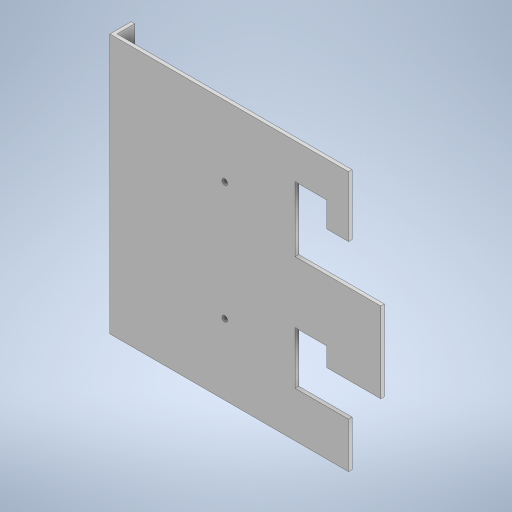
# Autodesk Inventor part: Coffee_Machine_Base
Saved by Autodesk Inventor 2023.5 (Build 275446020, 446B)
## iProperties
Created: 2025-04-17
Part Number: Coffee_Machine_Base
Material: Generic
Document SubType Name: Modeling
Designer: Lucky Sah
Density: 1 g/cm^3
Appearance: Default
Author: Lucky Sah
Autodesk Inventor part; units mm, degrees
ref_plane "YZ Plane" through (0, 0, 0) normal (1, 0, 0) x (0, 1, 0)
ref_plane "XZ Plane" through (0, 0, 0) normal (0, 1, 0) x (-1, 0, 0)
ref_plane "XY Plane" through (0, 0, 0) normal (0, 0, 1) x (1, 0, 0)
sketch "Sketch1" plane through (0, 0, 0) normal (0, 0, 1) x (1, 0, 0)
  line L0 (0, 0) -> (260, 0)
  line L1 (260, 0) -> (260, 125)
  line L2 (220, 147) -> (0, 147)
  line L3 (0, 147) -> (0, 0)
  circle A0 centre (240, 135) radius 8
  circle A1 centre (240, 135) radius 10
  line L4 (250, 135) -> (250.202, 135)
  line L5 (230, 135) -> (230, 137)
  arc A2 (230, 137) -> (220, 147) centre (220, 137) ccw
  line L6 (260, 147) -> (260, 147)
  line L7 (250, 135) -> (250, 137)
  line L8 (240, 125) -> (260, 125)
  line L9 (0, 73.5) -> (260, 73.5)
  line L10 (130, 112.7628) -> (117.7684, 112.7628)
  line L11 (99.8322, 119.3312) -> (99.8322, 90.3139)
  line L12 (99.8322, 90.3139) -> (148.259, 90.3139)
  line L13 (148.259, 90.3139) -> (148.259, 44.839)
  line L14 (148.259, 44.839) -> (117.7684, 44.839)
  line L15 (99.8322, 44.839) -> (99.8322, 25.7829)
  line L16 (99.8322, 25.7829) -> (130, 25.7829)
  line L17 (99.8322, 119.3312) -> (99.8322, 127)
  line L18 (99.8322, 127) -> (117.7684, 127)
  line L19 (117.7684, 127) -> (117.7684, 112.7628)
  line L20 (99.8322, 44.839) -> (99.8322, 55.475)
  line L21 (99.8322, 55.475) -> (117.7684, 55.475)
  line L22 (117.7684, 55.475) -> (117.7684, 44.839)
  line L23 (130, 147) -> (130, 112.7628)
  line L24 (130, 25.7829) -> (130, 0)
  line L25 (60, 107) -> (200, 107)
  line L26 (200, 107) -> (200, 40)
  line L27 (200, 40) -> (60, 40)
  line L28 (60, 40) -> (60, 107)
  circle A3 centre (60, 107) radius 1.5
  circle A4 centre (200, 107) radius 1.5
  circle A5 centre (200, 40) radius 1.5
  circle A6 centre (60, 40) radius 1.5
  circle A7 centre (130, 107) radius 1.5
  circle A8 centre (130, 40) radius 1.5
  line L29 (260, 125) -> (265, 125)
  line L30 (265, 0) -> (260, 0)
  line L31 (260, 0) -> (260, 125)
  line L32 (265, 0) -> (263, 0)
  line L33 (0, 147) -> (-3, 147)
  line L34 (-3, 147) -> (-3, 0)
  line L35 (-3, 0) -> (0, 0)
  line L36 (0, 0) -> (0, 147)
  line L37 (-3, 147) -> (-5, 147)
  line L38 (-5, 147) -> (-5, 0)
  line L39 (-5, 0) -> (-3, 0)
  line L40 (-3, 0) -> (-3, 147)
  point P0 (260, 67.5)
  point P1 (263, 125)
  point P2 (200, 73.5)
  point P3 (148.259, 73.5)
  point P4 (99.8322, 107)
  point P5 (128.5, 107)
  point P6 (131.5, 107)
  point P7 (198.5, 107)
  point P8 (200, 105.5)
  point P9 (60, 73.5)
  point P10 (99.8322, 40)
  dimension "d2" = 16
  dimension "d3" = 20
  dimension "d4" = 135
  dimension "d5" = 2
  dimension "d6" = 260
  dimension "d7" = 147
  dimension "d8" = 10
  dimension "d11" = 22
  dimension "d16" = 40
  dimension "d17" = 40
  dimension "d18" = 60
  dimension "d19" = 60
  dimension "d20" = 3
  dimension "d21" = 3
  dimension "d22" = 3
  dimension "d23" = 3
  dimension "d24" = 140
  dimension "d25" = 67
  dimension "d26" = 3
  dimension "d27" = 3
  dimension "d28" = 70
  dimension "d29" = 70
  dimension "d30" = 5
  dimension "d31" = 2
  dimension "d41" = 3
  dimension "d42" = 2
  constraints: 84 end point, 21 perpendicular, 15 point on line, 9 centre point, 9 parallel, 5 horizontal, 5 point on circle, 4 coincident, 4 midpoint, 4 tangent, 1 collinear
  measures "d2" diameter of A0
  measures "d3" distance from line of L1 A0.centre
  measures "d4" distance from line of L0 A0.centre
  measures "d5" radial gap between concentric circles of A0 A1
  measures "d6" distance from line of point (260, 67.5) L3
  measures "d7" distance between parallel lines of L0 L2
  measures "d8" radius of A2
  measures "d11" distance between parallel lines of L2 L8
  measures "d16" distance between parallel lines of L25 L2
  measures "d17" distance between parallel lines of L0 L27
  measures "d18" distance between parallel lines of L3 L28
  measures "d19" distance between parallel lines of L1 L26
  measures "d20" diameter of A3
  measures "d21" diameter of A4
  measures "d22" diameter of A5
  measures "d23" diameter of A6
  measures "d24" distance between parallel lines of L26 L28
  measures "d25" distance between parallel lines of L27 L25
  measures "d26" diameter of A7
  measures "d27" diameter of A8
  measures "d28" distance from line of L26 A7.centre
  measures "d29" distance from line of L26 A8.centre
  measures "d30" distance of L30.start L30.end
  measures "d31" distance of L30.start L32.end
  measures "d41" distance of L35.end L34.end
  measures "d42" distance of L39.end L38.end
extrude "Extrusion1" add sketch "Sketch1" along normal blind 2 contours L3 L9 L28 A6 L27 L15 L16 L24 L0 | L35 L34 L33 L3 | L3 L2 L23 L10 L19 L18 L17 L11 L25 A3 L28 L9 | L39 L38 L37 L34 | L28 A3 L25 L11 L12 L13 L9 | L9 L13 L14 L22 L21 L20 L15 L27 A6 L28
sketch "Sketch4" plane through (0, 0, 0) normal (0, 0, -1) x (-1, 0, 0)
  line L0 (-130, 147) -> (5, 147) projected
  line L1 (5, 0) -> (-130, 0) projected
  line L2 (5, 147) -> (3, 147)
  line L3 (3, 147) -> (3, 0)
  line L4 (3, 0) -> (5, 0)
  line L5 (5, 0) -> (5, 147)
  point P0 (0, 0)
  dimension "d43" = 2
  constraints: 8 end point, 2 parallel, 1 horizontal, 1 perpendicular, 1 point on line
  measures "d43" distance of L4.end L3.end
extrude "Extrusion4" add sketch "Sketch4" along normal blind 10
sketch "Sketch5" plane through (-5, 0, 2) normal (-1, 0, 0) x (0, 0, 1)
  line L0 (-12, 147) -> (-12, 0) projected
  line L1 (-2, 0) -> (-12, 0) projected
  line L2 (-12, 147) -> (-6, 147)
  line L3 (-6, 147) -> (-6, 0)
  line L4 (-6, 0) -> (-12, 0)
  line L5 (-12, 0) -> (-12, 147)
  circle A0 centre (-6, 127) radius 1.5
  circle A1 centre (-6, 20) radius 1.5
  line L6 (-12, 147) -> (0, 147) projected
  line L7 (-12, 0) -> (0, 0) projected
  point P0 (-6, 147)
  point P1 (-6, 0)
  dimension "d46" = 6
  dimension "d47" = 3
  dimension "d48" = 3
  dimension "d49" = 20
  dimension "d50" = 20
  constraints: 8 end point, 3 point on line, 2 centre point, 2 midpoint, 2 parallel, 1 horizontal, 1 perpendicular
  measures "d46" distance of L3.end L4.end
  measures "d47" diameter of A0
  measures "d48" diameter of A1
  measures "d49" distance of point (-6, 147) A0.centre
  measures "d50" distance of A1.centre point (-6, 0)
extrude "Extrusion5" cut sketch "Sketch5" against normal blind 10 contours A0 L3 | L3 A0 | A1 L3 | L3 A1
body "Solid1"
